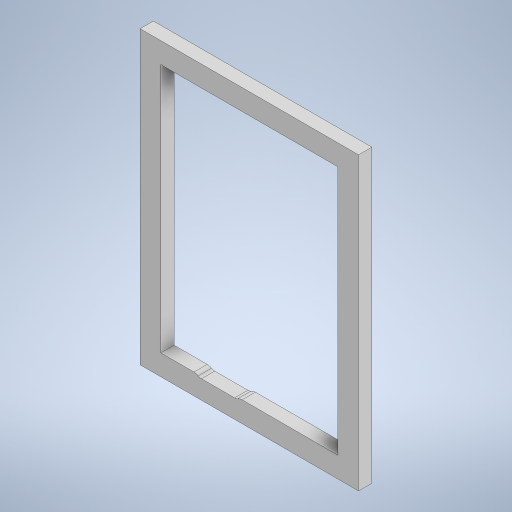
# Autodesk Inventor part: LCDFrame
Saved by Autodesk Inventor 2024 (Build 280153000, 153)
## iProperties
Created: 2023-10-07
Part Number: LCDFrame
Material: Generic
Document SubType Name: Modeling
Designer: chris
Density: 1 g/cm^3
Appearance: Default
Author: chris
Autodesk Inventor part; units mm, degrees
ref_plane "YZ Plane" through (0, 0, 0) normal (1, 0, 0) x (0, 1, 0)
ref_plane "XZ Plane" through (0, 0, 0) normal (0, 1, 0) x (-1, 0, 0)
ref_plane "XY Plane" through (0, 0, 0) normal (0, 0, 1) x (1, 0, 0)
sketch "Sketch1" plane through (0, 0, 0) normal (0, 0, 1) x (1, 0, 0)
  line L0 (-26.36, -35.13) -> (26.36, -35.13)
  line L1 (26.36, -35.13) -> (26.36, 35.13)
  line L2 (26.36, 35.13) -> (-26.36, 35.13)
  line L3 (-26.36, 35.13) -> (-26.36, -35.13)
  line L4 (-26.36, -35.13) -> (26.36, 35.13) construction
  line L5 (26.36, -35.13) -> (-26.36, 35.13) construction
  line L6 (-21.36, -30.13) -> (21.36, -30.13)
  line L7 (21.36, -30.13) -> (21.36, 30.13)
  line L8 (21.36, 30.13) -> (-21.36, 30.13)
  line L9 (-21.36, 30.13) -> (-21.36, -30.13)
  line L10 (-21.36, -30.13) -> (21.36, 30.13) construction
  line L11 (21.36, -30.13) -> (-21.36, 30.13) construction
  point P0 (0, 0)
  dimension "t" = 5
  dimension "d1" = 5
  dimension "d2" = 60.26
  dimension "d3" = 42.72
  constraints: 24 end point, 4 midpoint, 4 parallel, 2 horizontal, 2 perpendicular
  measures "t" distance between parallel lines of L2 L8
  measures "d1" distance between parallel lines of L1 L7
  measures "d2" distance between parallel lines of L6 L8
  measures "d3" distance between parallel lines of L7 L9
extrude "Extrusion1" add sketch "Sketch1" along normal blind 3.2
sketch "Sketch2" plane through (0, 0, 3.2) normal (0, 0, 1) x (1, 0, 0)
  line L0 (-11.5572, -30.63) -> (-3.5572, -30.63)
  arc A0 (-3.5572, -30.63) -> (-2.7846, -30.4157) centre (-3.5572, -29.13) ccw
  arc A1 (-1.7544, -30.13) -> (-2.7846, -30.4157) centre (-1.7544, -32.13) ccw
  line L1 (21.36, -30.13) -> (-21.36, -30.13) projected
  line L2 (-7.5572, -30.63) -> (-7.5572, -30.13)
  arc A2 (-12.3298, -30.4157) -> (-11.5572, -30.63) centre (-11.5572, -29.13) ccw
  arc A3 (-12.3298, -30.4157) -> (-13.36, -30.13) centre (-13.36, -32.13) ccw
  point P0 (0, 0)
  point P1 (-13.36, -30.13)
  dimension "d6" = 0.5
  dimension "d7" = 8
  dimension "d8" = 1.5
  dimension "d9" = 2
  dimension "d10" = 8
  constraints: 8 point on circle, 4 centre point, 4 end point, 4 symmetric about line, 3 tangent, 2 point on line, 1 horizontal, 1 midpoint, 1 perpendicular, 2 other
  measures "d6" distance between parallel lines of L1 L0
  measures "d7" distance of L0.start L0.end
  measures "d8" radius of A2
  measures "d9" radius of A3
  measures "d10" distance of L1.end A3.end
extrude "Extrusion2" cut sketch "Sketch2" against normal blind 3.2
equation "\"d1\" = t"
body "Solid1"
